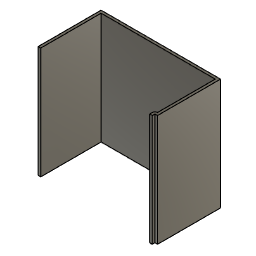
Vent Director Extender v2 (Autodesk Fusion 360 design; units mm, degrees)
Autodesk Fusion 360 part; units mm, degrees
sketch "Sketch1" plane through (0, 0, 0) normal (0, 0, 1) x (1, 0, 0)
  line L0 (0, 0) -> (0, -76.2)
  line L1 (0, -76.2) -> (3.175, -76.2)
  line L2 (3.175, -76.2) -> (3.175, -3.175)
  line L3 (0, 0) -> (144.4625, 0)
  line L4 (144.4625, 0) -> (144.4625, -76.2)
  line L5 (144.4625, -76.2) -> (141.2875, -76.2)
  line L6 (141.2875, -76.2) -> (141.2875, -3.175)
  line L7 (141.2875, -3.175) -> (3.175, -3.175)
  dimension "d1" = 76.2
  dimension "d2" = 3.175
  dimension "d3" = 73.025
  dimension "d4" = 144.4625
  dimension "d5" = 76.2
  dimension "d6" = 3.175
  dimension "d7" = 73.025
  constraint coincident L0.start L3.start
  constraint vertical L0
  constraint perpendicular L0 L1
  constraint perpendicular L1 L2
  constraint perpendicular L0 L3
  constraint perpendicular L3 L4
  constraint perpendicular L4 L5
  constraint perpendicular L5 L6
  measures "d1" distance of L0.start L0.end
  measures "d2" distance of L0.end L1.end
  measures "d3" distance of L1.end L2.end
  measures "d4" distance of L0.start L3.end
  measures "d5" distance of L3.end L4.end
  measures "d6" distance of L4.end L5.end
  measures "d7" distance of L5.end L6.end
extrude "Extrude1" add sketch "Sketch1" along normal blind 134.9375
sketch "Sketch2" plane through (141.2875, 0, 0) normal (-1, 0, 0) x (0, -1, 0)
  line L0 (3.175, 0) -> (76.2, 0)
  line L1 (76.2, 0) -> (76.2, 134.9375)
  line L2 (76.2, 134.9375) -> (3.175, 134.9375)
  line L3 (3.175, 134.9375) -> (3.175, 0)
  line L4 (76.2, 134.9375) -> (73.025, 134.9375)
  line L5 (73.025, 134.9375) -> (73.025, 0)
  line L6 (73.025, 0) -> (76.2, 0)
  line L7 (76.2, 0) -> (76.2, 134.9375)
  dimension "d11" = 3.175
  constraint horizontal L4
  constraint vertical L5
  constraint horizontal L6
  constraint vertical L7
  constraint coincident L1.end L2.start
  measures "d11" distance of L1.end L4.end
revolve "Revolve1" add sketch "Sketch2" angle 90 about axis through (141.2875, -76.2, 0) along (0, 0, 1) contours L0 L1 L2 L4 L5 L6 L7
sketch "Sketch3" plane through (0, -76.2, 0) normal (0, -1, 0) x (1, 0, 0)
  line L0 (138.1125, 0) -> (144.4625, 0)
  line L1 (144.4625, 0) -> (144.4625, 134.9375)
  line L2 (144.4625, 134.9375) -> (138.1125, 134.9375)
  line L3 (138.1125, 134.9375) -> (138.1125, 0)
  line L4 (138.1125, 134.9375) -> (141.2875, 134.9375)
  line L5 (141.2875, 134.9375) -> (141.2875, 0)
  line L6 (141.2875, 0) -> (138.1125, 0)
  line L7 (138.1125, 0) -> (138.1125, 134.9375)
  dimension "d13" = 3.175
  constraint horizontal L4
  constraint vertical L5
  constraint horizontal L6
  constraint vertical L7
  constraint coincident L2.end L3.start
  measures "d13" distance of L2.end L4.end
extrude "Extrude2" add sketch "Sketch3" along normal blind 3.175 contours L0 L2 L3 L4 L5 L6 L7
equation "Length = ( 10.625 / 2 ) * 1 in"
equation "d9 = Length"
